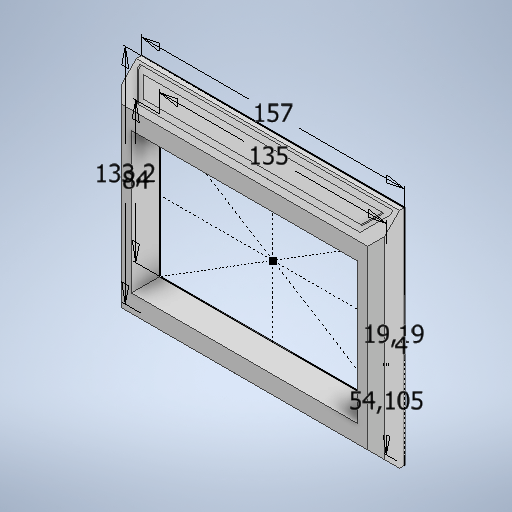
# Autodesk Inventor part: up_part
Saved by Autodesk Inventor 2025 (Build 290162000, 162)
## iProperties
Created: 2026-07-31
Part Number: up_part
Material: Типовые
Document SubType Name: Modeling
Designer: garin
Density: 1 g/cm^3
Appearance: По умолчанию
Author: garin
Autodesk Inventor part; units mm, degrees
ref_plane "YZ Plane" through (0, 0, 0) normal (1, 0, 0) x (0, 1, 0)
ref_plane "XZ Plane" through (0, 0, 0) normal (0, 1, 0) x (-1, 0, 0)
ref_plane "XY Plane" through (0, 0, 0) normal (0, 0, 1) x (1, 0, 0)
sketch "Эскиз1" plane through (0, 0, 0) normal (0, 0, 1) x (1, 0, 0)
  line L0 (0, 0) -> (-157, 0)
  line L1 (-157, 0) -> (-157, 133.2)
  line L2 (-157, 133.2) -> (0, 133.2)
  line L3 (0, 133.2) -> (0, 0)
  line L4 (-157, 66.6) -> (0, 66.6) construction
  line L5 (-78.5, 0) -> (-78.5, 133.2) construction
  line L6 (-11, 24.6) -> (-146, 24.6)
  line L7 (-146, 24.6) -> (-146, 108.6)
  line L8 (-146, 108.6) -> (-11, 108.6)
  line L9 (-11, 108.6) -> (-11, 24.6)
  line L10 (-11, 24.6) -> (-146, 108.6) construction
  line L11 (-146, 24.6) -> (-11, 108.6) construction
  line L12 (0, 0) -> (-4, 0) construction
  line L13 (-4, 0) -> (-4, 54.105) construction
  line L14 (-4, 54.105) -> (0, 54.105) construction
  line L15 (0, 54.105) -> (0, 0) construction
  line L16 (-4, 54.105) -> (-4, 73.295)
  line L17 (-4, 73.295) -> (-11, 73.295)
  line L18 (-4, 54.105) -> (-11, 54.105)
  point P0 (-78.5, 66.6)
  dimension "d0" = 157
  dimension "d1" = 133.2
  dimension "d2" = 135
  dimension "d3" = 84
  dimension "d20" = 4
  dimension "d21" = 54.105
  dimension "d22" = 19.19
  constraints: 38 end point, 7 midpoint, 6 parallel, 5 perpendicular, 3 horizontal, 2 point on line, 1 vertical
  measures "d0" distance of L1.end L2.end
  measures "d1" distance of L0.end L1.end
  measures "d2" distance of L7.end L8.end
  measures "d3" distance of L6.end L7.end
  measures "d20" distance of L13.end L14.end
  measures "d21" distance of L12.end L13.end
  measures "d22" distance of L13.end L16.end
extrude "Выдавливание1" add sketch "Эскиз1" along normal blind 17 contours L0 L1 L2 L3 | L9 L17 L16 L18
chamfer "Фаска1" distance 14 angle 45 2 edges at (-78.5, 0, 17) (-78.5, 133.2, 17)
chamfer "Фаска2" distance 5 angle 45 2 edges at (-157, 66.6, 17) (0, 66.6, 17)
sketch "Эскиз2" plane through (-157, 0, 3) normal (0, -0.7071068, 0.7071068) x (1, 0, 0)
  line L0 (0, -2.1213) -> (157, -2.1213) projected
  line L1 (0, -2.1213) -> (157, -2.1213)
  line L2 (157, -2.1213) -> (157, 19.7987)
  line L3 (157, 19.7987) -> (0, 19.7987)
  line L4 (0, 19.7987) -> (0, -2.1213)
  line L5 (78.5, 19.7987) -> (78.5, -2.1213) construction
  line L6 (0, 8.8387) -> (157, 8.8387) construction
  line L7 (154, 1.3387) -> (3, 1.3387) construction
  line L8 (3, 1.3387) -> (3, 16.3387) construction
  line L9 (3, 16.3387) -> (154, 16.3387) construction
  line L10 (154, 16.3387) -> (154, 1.3387) construction
  line L11 (154, 1.3387) -> (3, 16.3387) construction
  line L12 (3, 1.3387) -> (154, 16.3387) construction
  line L13 (3, 16.3387) -> (12, 16.3387) construction
  line L14 (12, 16.3387) -> (3, 3.6108)
  line L15 (0, 12.7279) -> (5, 19.799) construction
  line L16 (145, 16.3387) -> (154, 3.6108)
  line L17 (12, 16.3387) -> (145, 16.3387)
  line L18 (11, 15.2735) -> (11, 27.2943) projected
  line L19 (154, 3.6108) -> (154, 1.3387)
  line L20 (154, 1.3387) -> (3, 1.3387)
  line L21 (3, 3.6108) -> (3, 1.3387)
  line L22 (7.189, 4.3387) -> (13.5529, 13.3387)
  line L23 (13.5529, 13.3387) -> (143.4471, 13.3387)
  line L24 (143.4471, 13.3387) -> (149.811, 4.3387)
  line L25 (149.811, 4.3387) -> (7.189, 4.3387)
  point P0 (78.5, 8.8387)
  dimension "d12" = 157
  dimension "d13" = 21.92
  dimension "d14" = 151
  dimension "d15" = 15
  dimension "d16" = 9
  dimension "d17" = 3
  constraints: 46 end point, 7 midpoint, 5 parallel, 5 perpendicular, 2 horizontal, 2 point on line, 2 symmetric about line, 1 collinear, 3 other
  measures "d12" distance of L3.end L2.end
  measures "d13" distance of L2.end L1.end
  measures "d14" distance of L8.end L9.end
  measures "d15" distance of L7.end L8.end
  measures "d16" distance of L8.end L13.end
  measures "d17" distance between parallel lines of L14 L22
extrude "Выдавливание2" cut sketch "Эскиз2" against normal blind 1.2 contours L17 L16 L19 L20 L21 L14
ref_plane "РабПлоскость1" through (-157, 66.6, 0) normal (0, 1, 0) x (1, 0, 0)
mirror "Зеркальное отражение1" about plane through (-157, 66.6, 0) normal (0, 1, 0) of "Выдавливание2"
extrude "Выдавливание3" cut sketch "Эскиз1" along normal blind 15 contours L9 L17 L16 L18
